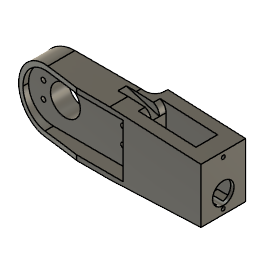
Link2 (Autodesk Fusion 360 design; units mm, degrees)
part number: 2026-06-19-16-40-55-659
Autodesk Fusion 360 part; units mm, degrees
note: some values were not read from the file. Chosen so that the rebuilt part matches the saved one: which face or edge a step refers to. Set by a fixed rule: which sketch regions a step uses.
sketch "Sketch1" plane through (0, 0, 0) normal (0, 1, 0) x (1, 0, 0)
  line L0 (60, 19) -> (-60, 19)
  line L1 (-60, 19) -> (-60, -19)
  line L2 (-60, -19) -> (60, -19)
  line L3 (60, -19) -> (60, 19)
  line L4 (60, 19) -> (-60, -19) construction
  line L5 (-60, 19) -> (60, -19) construction
  line L6 (-4, 10.5) -> (-45, 10.5)
  line L7 (-45, 10.5) -> (-45, -10.5)
  line L8 (-45, -10.5) -> (-4, -10.5)
  line L9 (-4, -10.5) -> (-4, 10.5)
  line L10 (-4, 10.5) -> (-45, -10.5) construction
  line L11 (-45, 10.5) -> (-4, -10.5) construction
  point P0 (-24.5, 0)
  dimension "d1" = 120
  dimension "d2" = 38
  dimension "d3" = 8.5
  dimension "d4" = 21
  dimension "d5" = 15
  dimension "d6" = 41
  constraint horizontal L0
  constraint perpendicular L0 L1
  constraint parallel L0 L2
  constraint parallel L1 L3
  constraint coincident L4 origin
  constraint coincident L5 origin
  constraint horizontal L6
  constraint perpendicular L6 L7
  constraint parallel L6 L8
  constraint parallel L7 L9
  constraint coincident L10 P0
  constraint coincident L11 P0
  measures "d1" distance of L1.end L2.end
  measures "d2" distance of L0.start L2.end
  measures "d3" distance of L2 L8
  measures "d4" distance of L6.end L7.end
  measures "d5" distance of L1 L7
  measures "d6" distance of L6.start L6.end
extrude "Extrude1" add sketch "Sketch1" along normal blind 11
fillet "Fillet1" radius 20 1 edges at (-60, 5.5, 19)
fillet "Fillet2" radius 18 3 edges at (-60, 0, -10) (-60, 11, -10) (-60, 5.5, -19)
sketch "Sketch2" plane through (0, 0, 0) normal (0, -1, 0) x (1, 0, 0)
  arc A0 (-60, -1) -> (-42, -19) centre (-42, -1) ccw
  line L0 (-42, -19) -> (60, -19)
  line L1 (60, -19) -> (60, 19)
  line L2 (60, 19) -> (-40, 19)
  arc A1 (-40, 19) -> (-60, -1) centre (-40, -1) ccw
  line L3 (-4, 10.5) -> (-4, -10.5)
  line L4 (-4, -10.5) -> (-45, -10.5)
  line L5 (-45, -10.5) -> (-45, 10.5)
  line L6 (-45, 10.5) -> (-4, 10.5)
  line L7 (57, 16) -> (-40, 16)
  arc A2 (-40, 16) -> (-57, -1) centre (-40, -1) ccw
  arc A3 (-57, -1) -> (-42, -16) centre (-42, -1) ccw
  line L8 (-42, -16) -> (57, -16)
  line L9 (57, -16) -> (57, 16)
  dimension "d11" = -3
extrude "Extrude2" add sketch "Sketch2" along normal blind 8 contours A0 L0 L1 L2 A1
sketch "Sketch3" plane through (0, 0, 0) normal (0, 0, 1) x (1, 0, 0)
  line L0 (-60, 11) -> (-60, -8)
  line L1 (-60, -8) -> (-40, -8)
  line L2 (-40, 11) -> (-40, -8)
  line L3 (-40, -8) -> (60, -8)
  line L4 (60, -8) -> (60, 11)
  line L5 (60, 11) -> (-40, 11)
  line L6 (-60, -3) -> (-60, -8)
  line L7 (-60, -8) -> (-20, -8)
  spline S0 degree 5 poles (-60, -3) (-59.0082, -3.1148) (-57.0406, -3.3431) (-54.1366, -3.6819) (-50.3613, -4.1261) (-45.8151, -4.6682) (-41.4598, -5.1955) (-37.3159, -5.7066) (-33.4012, -6.2) (-29.7202, -6.6755) (-26.2611, -7.1338) (-23.6596, -7.4878) (-21.7962, -7.7465) (-20.5923, -7.916) (-20, -8) knots 0 0 0 0 0 0 0.1 0.2 0.3 0.4 0.5 0.6 0.7 0.8 0.9 1 1 1 1 1 1
  point P0 (-35, -6)
  dimension "d14" = 5
  dimension "d15" = 40
  dimension "d16" = 25
  dimension "d17" = 2
  constraint coincident L0 L6.start
  constraint coincident L0.end L1.start
  constraint coincident L3 L7.end
  measures "d14" distance of L6.start L0.end
  measures "d15" distance of L0.end L7.end
  measures "d16" horizontal distance of L6.start P0
  measures "d17" distance of L7 P0
extrude "Extrude3" cut sketch "Sketch3" along normal mid plane 66 contours L0 L1 L2 L6 L7 S0 | L2 L3 L7 S0
sketch "Sketch4" plane through (0, 0, 0) normal (0, -1, 0) x (1, 0, 0)
  line L0 (57, 16) -> (-40, 16)
  arc A0 (-40, 16) -> (-57, -1) centre (-40, -1) ccw
  arc A1 (-57, -1) -> (-42, -16) centre (-42, -1) ccw
  line L1 (-42, -16) -> (57, -16)
  line L2 (57, -16) -> (57, 16)
  line L3 (-4, 10.5) -> (-4, -10.5)
  line L4 (-4, -10.5) -> (-45, -10.5)
  line L5 (-45, -10.5) -> (-45, 10.5)
  line L6 (-45, 10.5) -> (-4, 10.5)
  line L7 (-20, -16) -> (-20, -19)
  line L8 (-20, -19) -> (60, -19)
  line L9 (60, -19) -> (60, 19)
  line L10 (60, 19) -> (-20, 19)
  line L11 (-20, 19) -> (-20, 16)
  line L12 (-20, 16) -> (57, 16)
  line L13 (57, 16) -> (57, -16)
  line L14 (57, -16) -> (-20, -16)
  line L15 (57, 16) -> (8, 16)
  line L16 (8, 16) -> (8, -16)
  line L17 (8, -16) -> (57, -16)
  line L18 (57, -16) -> (57, 16)
  dimension "d20" = 49
  constraint horizontal L15
  constraint vertical L16
  constraint horizontal L17
  constraint vertical L18
  constraint coincident L14 L16.end
  constraint coincident L0.start L2.end
  measures "d20" distance of L16.end L1.end
extrude "Extrude4" add sketch "Sketch4" along normal up to surface (8 mm away) contours L0 L1 L2 L12 L13 L14 L15 L16 L17 L18
sketch "Sketch5" plane through (0, 11, 0) normal (0, 1, 0) x (-1, 0, 0)
  line L0 (4, -10.5) -> (4, 10.5)
  line L1 (4, 10.5) -> (45, 10.5)
  line L2 (45, 10.5) -> (45, -10.5)
  line L3 (45, -10.5) -> (4, -10.5)
  arc A0 (42, -19) -> (60, -1) centre (42, -1) ccw
  arc A1 (60, -1) -> (40, 19) centre (40, -1) ccw
  line L4 (40, 19) -> (-60, 19)
  line L5 (-60, 19) -> (-60, -19)
  line L6 (-60, -19) -> (42, -19)
  line L7 (-60, 19) -> (-8, 19)
  line L8 (-8, 19) -> (-8, -19)
  line L9 (-8, -19) -> (-60, -19)
  line L10 (-60, -19) -> (-60, 19)
  dimension "d23" = 52
  constraint horizontal L7
  constraint vertical L8
  constraint horizontal L9
  constraint vertical L10
  constraint coincident L6 L8.end
  constraint coincident L4.end L5.start
  measures "d23" distance of L8.end L5.end
extrude "Extrude5" add sketch "Sketch5" along normal blind 8 contours L4 L5 L6 L7 L8 L9 L10
extrude "Extrude6" cut 1 faces at (60, 10, 6.3333) along direction (-1, 0, 0) blind 5
sketch "Sketch6" plane through (0, 0, -19) normal (0, 0, -1) x (1, 0, 0)
  line L0 (55, -19) -> (55, 8)
  line L1 (55, 8) -> (-20, 8)
  spline S0 degree 3 poles (-20, 8) (-27.1586, 6.9847) (-34.5551, 6.0398) (-42, 5.132) knots 0 0 0 0 2.169078 2.169078 2.169078 2.169078
  line L2 (-42, 5.132) -> (-42, -11)
  line L3 (-42, -11) -> (8, -11)
  line L4 (8, -11) -> (8, -19)
  line L5 (8, -19) -> (55, -19)
  line L6 (45, 1) -> (14, 1)
  line L7 (14, 1) -> (14, -12)
  line L8 (14, -12) -> (45, -12)
  line L9 (45, -12) -> (45, 1)
  dimension "d28" = 10
  dimension "d29" = 7
  dimension "d30" = 31
  dimension "d31" = 13
  constraint horizontal L6
  constraint vertical L7
  constraint horizontal L8
  constraint vertical L9
  measures "d28" horizontal distance of L0.end L6.start
  measures "d29" distance of L1 L6
  measures "d30" distance of L6.start L6.end
  measures "d31" distance of L6.start L8.end
extrude "Extrude7" cut sketch "Sketch6" against normal blind 40 contours L6 L7 L8 L9
sketch "Sketch7" plane through (0, 11, 0) normal (0, 1, 0) x (-1, 0, 0)
  line L0 (-8, 19) -> (-8, -19)
  line L1 (-8, -19) -> (42, -19)
  arc A0 (42, -19) -> (60, -1) centre (42, -1) ccw
  arc A1 (60, -1) -> (40, 19) centre (40, -1) ccw
  line L2 (40, 19) -> (-8, 19)
  line L3 (4, -10.5) -> (4, 10.5)
  line L4 (4, 10.5) -> (45, 10.5)
  line L5 (45, 10.5) -> (45, -10.5)
  line L6 (45, -10.5) -> (4, -10.5)
  circle A2 centre (34.75, 1) radius 9
  dimension "d34" = 18
  dimension "d35" = 10.25
  measures "d34" diameter of A2
  measures "d35" horizontal distance of L5.end A2.centre
extrude "Extrude8" add sketch "Sketch7" against normal up to surface (11 mm away) contours L3 L4 L5 L6
sketch "Sketch8" plane through (45, 0, 0) normal (-1, 0, 0) x (0, -1, 0)
  line L0 (1, 19) -> (-12, 19)
  line L1 (-12, 19) -> (-12, -19)
  line L2 (-12, -19) -> (1, -19)
  line L3 (1, -19) -> (1, 19)
  line L4 (1, 0) -> (-12, 0) construction
  line L5 (-12, 11.5) -> (1, 11.5)
  line L6 (1, 11.5) -> (1, -11.5)
  line L7 (1, -11.5) -> (-12, -11.5)
  line L8 (-12, -11.5) -> (-12, 11.5)
  line L9 (-12, 11.5) -> (1, -11.5) construction
  line L10 (1, 11.5) -> (-12, -11.5) construction
  point P0 (-5.5, 0)
  dimension "d38" = 7.5
  constraint midpoint L3 L4.start
  constraint midpoint L1 L4.end
  constraint horizontal L5
  constraint perpendicular L5 L6
  constraint parallel L5 L7
  constraint parallel L6 L8
  constraint coincident L9 P0
  constraint coincident L10 P0
  constraint coincident L1 L5.start
  constraint midpoint L4 P0
  measures "d38" distance of L2 L7
extrude "Extrude9" cut sketch "Sketch8" against normal blind 8 contours L1 L3 L5 L6 L7 L8
sketch "Sketch9" plane through (14, 0, 0) normal (1, 0, 0) x (0, 1, 0)
  line L0 (12, 19) -> (-1, 19)
  line L1 (-1, 19) -> (-1, -19)
  line L2 (-1, -19) -> (12, -19)
  line L3 (12, -19) -> (12, 19)
  line L4 (5.5, 19) -> (5.5, -19) construction
  line L5 (3, 19) -> (8, 19)
  line L6 (8, 19) -> (8, 13)
  line L7 (8, 13) -> (3, 13)
  line L8 (3, 13) -> (3, 19)
  line L9 (-1, 0) -> (12, 0) construction
  line L10 (8, -13) -> (3, -13)
  line L11 (8, -19) -> (8, -13)
  line L12 (3, -13) -> (3, -19)
  line L13 (3, -19) -> (8, -19)
  point P0 (5.5, 13)
  dimension "d41" = 5
  dimension "d42" = 6
  constraint midpoint L0 L4.start
  constraint midpoint L2 L4.end
  constraint horizontal L5
  constraint vertical L6
  constraint horizontal L7
  constraint vertical L8
  constraint coincident L0 L5.start
  constraint midpoint L7 P0
  constraint coincident L4 P0
  constraint midpoint L1 L9.start
  constraint midpoint L3 L9.end
  constraint symmetric L5.start L9 L12.end
  constraint symmetric L5.end L9 L11.start
  constraint symmetric L6.end L9 L10.start
  constraint symmetric L7.end L9 L10.end
  measures "d41" distance of L5.start L5.end
  measures "d42" distance of L5.end L6.end
extrude "Extrude10" cut sketch "Sketch9" against normal blind 20 contours L0 L5 L6 L7 L8 | L2 L10 L11 L12 L13
chamfer "Chamfer1" distance 20 distance2 6 1 edges at (-6, 5.5, 13) measured on face at (7.3333, 6.3333, 13)
chamfer "Chamfer1" distance 20 distance2 6 1 edges at (-6, 5.5, -13) measured on face at (7.3333, 6.3333, -13)
fillet "Fillet3" radius 6 4 edges at (14, 1, 19) (14, 10, 19) (14, 1, -19) (14, 10, -19)
fillet "Fillet4" radius 6 1 edges at (8, 11, 0)
sketch "Sketch10" plane through (45, 0, 0) normal (-1, 0, 0) x (0, -1, 0)
  line L0 (-12, 11.5) -> (1, 11.5)
  line L1 (1, 11.5) -> (1, 19)
  line L2 (1, 19) -> (-12, 19)
  line L3 (-12, 19) -> (-12, 11.5)
  line L4 (8, -19) -> (-19, -19)
  line L5 (-19, -19) -> (-19, 19)
  line L6 (-19, 19) -> (8, 19)
  line L7 (8, 19) -> (8, -19)
  line L8 (-5.5, 19) -> (-5.5, -19) construction
  circle A0 centre (-5.5, 13.5) radius 1.1
  line L9 (-5.5, 0) -> (8, 0) construction
  circle A1 centre (-5.5, -13.5) radius 1.1
  dimension "d53" = 2.2
  dimension "d54" = 27
  constraint midpoint L6 L8.start
  constraint midpoint L4 L8.end
  constraint coincident L8 A0.centre
  constraint midpoint L8 L9.start
  constraint midpoint L7 L9.end
  constraint symmetric A0 L9 A1
  measures "d53" diameter of A0
  measures "d54" distance of A0.centre A1.centre
extrude "Extrude11" cut sketch "Sketch10" against normal blind 35 contours A0 | A1
sketch "Sketch11" plane through (0, -8, 0) normal (0, -1, 0) x (1, 0, 0)
  line L0 (55, -19) -> (55, 19)
  line L1 (55, 19) -> (-20, 19)
  line L2 (-20, 19) -> (-20, 16)
  line L3 (-20, 16) -> (8, 16)
  line L4 (8, 16) -> (8, -16)
  line L5 (8, -16) -> (-20, -16)
  line L6 (-20, -16) -> (-20, -19)
  line L7 (-20, -19) -> (55, -19)
  line L8 (55, 0) -> (-75, 0) construction
  line L9 (55, 19) -> (0, 19)
  line L10 (0, 19) -> (55, 16.5)
  line L11 (55, 19) -> (55, 16.5)
  line L12 (-0.005, 0) -> (-0.005, 5) construction
  line L13 (-0.005, 5) -> (-48.005, 5)
  line L14 (-48.005, 5) -> (-48.005, -5)
  line L15 (-48.005, -5) -> (-0.005, -5)
  line L16 (-0.005, -5) -> (-0.005, 5)
  circle A0 centre (-0.005, 5) radius 1.4
  circle A1 centre (-0.005, -5) radius 1.4
  circle A2 centre (-48.005, 5) radius 1.4
  circle A3 centre (-48.005, -5) radius 1.4
  line L17 (0, -19) -> (55, -16.5)
  line L18 (55, -19) -> (0, -19)
  line L19 (55, -19) -> (55, -16.5)
  point P0 (-0.005, 0)
  dimension "d57" = 2.5
  dimension "d58" = 55
  dimension "d60" = 48
  dimension "d61" = 10
  dimension "d62" = 2.8
  dimension "d63" = 2.8
  dimension "d64" = 2.8
  dimension "d65" = 2.8
  constraint midpoint L0 L8.start
  constraint perpendicular L0 L8
  constraint coincident L0.end L1.start
  constraint coincident L1 L9.end
  constraint coincident L0 L10.end
  constraint perpendicular L8 L12
  constraint horizontal L13
  constraint vertical L14
  constraint horizontal L15
  constraint vertical L16
  constraint coincident L8 P0
  constraint midpoint L16 P0
  constraint coincident P0 L12.start
  constraint coincident L12.end L13.start
  constraint coincident L15.end L16.start
  constraint coincident L13.end L14.start
  constraint coincident L14.end L15.start
  constraint symmetric L8 L0.end L0.start
  constraint symmetric L8 L9.end L17.start
  constraint symmetric L8 L10.end L17.end
  measures "d57" distance of L0.end L10.end
  measures "d58" distance of L0.end L9.end
  measures "d60" distance of L14.end L15.end
  measures "d61" distance of L13 L15
  measures "d62" diameter of A0
  measures "d63" diameter of A1
  measures "d64" diameter of A2
  measures "d65" diameter of A3
extrude "Extrude12" cut sketch "Sketch11" against normal blind 38 contours L0 L7 L17 L18 L19 | L0 L1 L9 L10 L11 | L13 L14 A2 | L13 L14 A2 | L13 L16 A0 | L13 L16 A0 | L14 L15 A3 | L14 L15 A3 | L15 L16 A1 | L15 L16 A1
sketch "Sketch12" plane through (55, 0, 0) normal (1, 0, 0) x (0, 1, 0)
  circle A0 centre (5.5, -13.5) radius 1.1
  circle A1 centre (5.5, 13.5) radius 1.1
  line L0 (19, 16.5) -> (-8, 16.5)
  line L1 (-8, 16.5) -> (-8, -16.5)
  line L2 (-8, -16.5) -> (19, -16.5)
  line L3 (19, -16.5) -> (19, 16.5)
  circle A2 centre (5.5, -5.3) radius 6.5
  dimension "d68" = 13
  dimension "d69" = 13.5
  dimension "d70" = 5.3
  measures "d68" diameter of A2
  measures "d69" distance of L3 A2.centre
  measures "d70" vertical distance of origin A2.centre
extrude "Extrude13" cut sketch "Sketch12" against normal up to surface (10 mm away) contours A2
